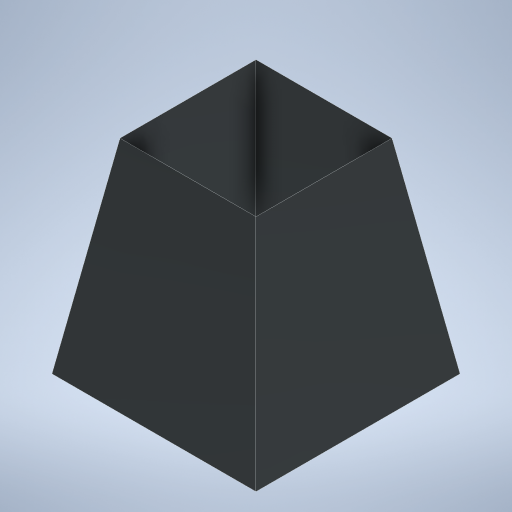
# Autodesk Inventor part: PostBase
Saved by Autodesk Inventor 2024.2 (Build 282272000, 272)
## iProperties
Created: 2024-01-23
Part Number: PostBase
Material: Iron, Cast
Document SubType Name: Modeling
Designer: airso
Density: 7.15 g/cm^3
Appearance: Iron Gray
Author: airso
Autodesk Inventor part; units mm, degrees
ref_plane "YZ Plane" through (0, 0, 0) normal (1, 0, 0) x (0, 1, 0)
ref_plane "XZ Plane" through (0, 0, 0) normal (0, 1, 0) x (-1, 0, 0)
ref_plane "XY Plane" through (0, 0, 0) normal (0, 0, 1) x (1, 0, 0)
sketch "Sketch1" plane through (0, 0, 0) normal (0, 1, 0) x (-1, 0, 0)
  line L0 (-50.8, 50.8) -> (50.8, 50.8)
  line L1 (50.8, 50.8) -> (50.8, -50.8)
  line L2 (50.8, -50.8) -> (-50.8, -50.8)
  line L3 (-50.8, -50.8) -> (-50.8, 50.8)
  line L4 (-50.8, 50.8) -> (50.8, -50.8) construction
  line L5 (50.8, 50.8) -> (-50.8, -50.8) construction
  line L6 (76.2, -76.2) -> (76.2, 76.2)
  line L7 (76.2, 76.2) -> (-76.2, 76.2)
  line L8 (-76.2, 76.2) -> (-76.2, -76.2)
  line L9 (-76.2, -76.2) -> (76.2, -76.2)
  point P0 (0, 0)
  dimension "d0" = 101.6
  dimension "d1" = 101.6
  dimension "d2" = 25.4
  constraints: 20 end point, 4 parallel, 2 midpoint, 2 perpendicular, 1 horizontal, 3 other
  measures "d0" distance of L1.end L2.end
  measures "d1" distance of L0.end L1.end
  measures "d2" distance between parallel lines of L1 L6
extrude "Extrusion1" add sketch "Sketch1" along normal blind 152.4
chamfer "Chamfer1" distance 25.4 distance2 152.4 1 edges at (0, 152.4, 76.2) measured on face at (-16.9333, 152.4, -67.7333)
chamfer "Chamfer2" distance 25.4 distance2 152.4 1 edges at (76.2, 152.4, -12.6998) measured on face at (-16.9333, 152.4, -67.7333)
chamfer "Chamfer3" distance 25.4 distance2 152.4 1 edges at (-12.6998, 152.4, -76.2) measured on face at (-25.3998, 152.4, -67.7333)
chamfer "Chamfer4" distance 25.4 distance2 152.4 1 edges at (-76.2, 152.4, 0) measured on face at (-67.7333, 152.4, -16.9333)
body "Solid1"
